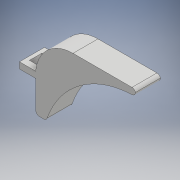
# Autodesk Inventor part: Positioner_Adapter
Saved by Autodesk Inventor 2018 (Build 220112000, 112)
## iProperties
Created: 2017-10-10
Part Number: Positioner_Adapter
Material: Genérico
Document SubType Name: Modeling
Designer: se_ma
Density: 1 g/cm^3
Appearance: Valor por defecto
Author: se_ma
Autodesk Inventor part; units mm, degrees
ref_plane "YZ Plane" through (0, 0, 0) normal (1, 0, 0) x (0, 1, 0)
ref_plane "XZ Plane" through (0, 0, 0) normal (0, 1, 0) x (-1, 0, 0)
ref_plane "XY Plane" through (0, 0, 0) normal (0, 0, 1) x (1, 0, 0)
sketch "Boceto1" plane through (0, 0, 0) normal (0, 1, 0) x (-1, 0, 0)
  line L0 (80, 80) -> (0, 80)
  line L1 (0, 80) -> (0, 75)
  line L2 (80, 47.68) -> (80, 52.68)
  line L3 (80, 47.68) -> (80, 22.68)
  line L4 (80, 22.68) -> (75, 22.68)
  line L5 (75, 22.68) -> (71.4886, 22.68)
  line L6 (80, 80) -> (80, 52.68)
  arc A0 (71.4886, 22.68) -> (0, 75) centre (0, 0) ccw
  dimension "d4" = 5
  dimension "d5" = 25
  constraints: 14 end point, 2 point on circle, 1 centre point, 1 coincident, 1 horizontal, 1 perpendicular, 1 vertical
  measures "d4" distance of L2.start L2.end
  measures "d5" distance of L2.start L3.end
extrude "Extrusión1" add sketch "Boceto1" along normal blind 20
sketch "Boceto2" plane through (-80, 0, 22.68) normal (-1, 0, 0) x (0, 0, 1)
  line L0 (0, 0) -> (52.32, 0) projected
  line L1 (25, 0) -> (30, 0)
  line L2 (30, 0) -> (30, 20)
  line L3 (0, 20) -> (52.32, 20) projected
  line L4 (25, 0) -> (25, 20)
  line L5 (25, 20) -> (30, 20)
  point P0 (-22.68, 0)
  dimension "d8" = 47.68
  dimension "d9" = 5
  constraints: 8 end point, 3 point on line, 1 collinear, 1 perpendicular, 1 vertical
  measures "d8" distance of point (-22.68, 0) L1.start
  measures "d9" distance of L1.start L1.end
extrude "Extrusión2" add sketch "Boceto2" along normal blind 13
sketch "Boceto3" plane through (-80, 0, 47.68) normal (0, 0, -1) x (-1, 0, 0)
  line L0 (0, 0) -> (13, 0) projected
  line L1 (0, 0) -> (3, 0)
  line L2 (0, 20) -> (13, 20) projected
  line L3 (3, 15) -> (10, 15)
  line L4 (10, 15) -> (10, 5)
  line L5 (10, 5) -> (3, 5)
  line L6 (3, 5) -> (3, 15)
  point P0 (-80, 0)
  dimension "d12" = 3
  dimension "d14" = 7
  dimension "d15" = 10
  constraints: 10 end point, 2 perpendicular, 1 point on line
  measures "d12" distance of L0.start L1.end
  measures "d14" distance of L3.start L3.end
  measures "d15" distance of L3.end L4.end
extrude "Extrusión3" cut sketch "Boceto3" against normal blind 5
fillet "Empalme1" radius 30 1 edges at (-80, 10, 80)
fillet "Empalme2" radius 3 4 edges at (-80, 10, 22.68) (-71.4886, 10, 22.68) (0, 10, 75) (0, 10, 80)
